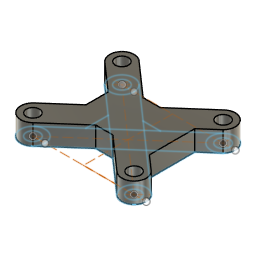
Drone v0 (Autodesk Fusion 360 design; units mm, degrees)
Autodesk Fusion 360 part; units mm, degrees
sketch "Skizze1" plane through (0, 0, 0) normal (0, 0, 1) x (1, 0, 0)
  line L0 (-50, 40) -> (0, 40) construction
  circle A0 centre (-50, 40) radius 3.25
  circle A1 centre (0, 40) radius 3.25
  line L1 (-25, 40) -> (-25, -4) construction
  line L2 (-25, -4) -> (0, -4) construction
  line L3 (0, -4) -> (-50, -4) construction
  circle A2 centre (-50, -4) radius 3.25
  circle A3 centre (0, -4) radius 3.25
  circle A4 centre (-50, 40) radius 6
  circle A5 centre (0, 40) radius 6
  circle A6 centre (0, -4) radius 6
  circle A7 centre (-50, -4) radius 6
  line L4 (-50, -4) -> (0, 40) construction
  line L5 (0, -4) -> (-50, 40) construction
  line L6 (-50, 40) -> (-50, 46) construction
  line L7 (-50, 40) -> (-49.8093, 40.2167) construction
  line L8 (-50, 40) -> (-45.7574, 44.2426) construction
  line L9 (-50, 40) -> (-44, 40) construction
  line L10 (-50, 40) -> (-56, 40) construction
  line L11 (-50, 40) -> (-54.2426, 35.7574) construction
  line L12 (0, -4) -> (6, -4) construction
  line L13 (0, -4) -> (4.2426, 0.2426) construction
  line L14 (0, -4) -> (6, -4) construction
  line L15 (0, -4) -> (0, -10) construction
  line L16 (0, -4) -> (-4.2426, -8.2426) construction
  line L17 (-4.2426, -8.2426) -> (-54.2426, 35.7574)
  line L18 (4.2426, 0.2426) -> (-45.7574, 44.2426)
  line L19 (0, 40) -> (0, 46) construction
  line L20 (0, 40) -> (-4.2426, 44.2426) construction
  line L21 (0, 40) -> (4.2426, 35.7574) construction
  line L22 (0, 40) -> (6, 40) construction
  line L23 (-50, -4) -> (-45.7574, -8.2426) construction
  line L24 (-50, -4) -> (-44, -4) construction
  line L25 (-50, -4) -> (-54.2426, 0.2426) construction
  line L26 (-50, -4) -> (-44, -4) construction
  line L27 (-54.2426, 0.2426) -> (-4.2426, 44.2426)
  line L28 (4.2426, 35.7574) -> (-45.7574, -8.2426)
  line L29 (-3.2166, 6.8068) -> (-3.2166, 29.1932)
  line L30 (-40.3073, 12.5057) -> (-40.3073, 23.4943)
  line L31 (-20.7574, 6.2903) -> (-29.2426, 6.2903)
  line L32 (-20.7574, 29.7097) -> (-29.2426, 29.7097)
  dimension "d2" = 6.5
  dimension "d3" = 6.5
  dimension "d4" = 6.5
  dimension "d5" = 6.5
  dimension "d6" = 12
  dimension "d7" = 12
  dimension "d8" = 12
  dimension "d9" = 45
  dimension "d10" = 135
  dimension "d11" = 6
  dimension "d12" = 45
  dimension "d13" = 135
  dimension "d14" = 135
  dimension "d15" = 45
  dimension "d16" = 6
  dimension "d17" = 45
  dimension "d18" = 135
  constraint horizontal L0
  constraint coincident L0.start A0.centre
  constraint coincident L0.end A1.centre
  constraint midpoint L0 L1.start
  constraint perpendicular L0 L1
  constraint perpendicular L1 L2
  constraint perpendicular L1 L3
  constraint coincident L3.end A2.centre
  constraint coincident L2.end L3.start
  constraint concentric A0 A4
  constraint concentric A1 A5
  constraint concentric A3 A6
  constraint concentric A2 A7
  constraint coincident A4 L6.end
  constraint vertical L6
  constraint perpendicular L5 L7
  constraint horizontal L9
  constraint coincident A4 L10.end
  constraint horizontal L10
  constraint coincident A6 L12.end
  constraint parallel L2 L12
  constraint horizontal L14
  constraint coincident A6 L15.end
  constraint vertical L15
  constraint coincident A5 L19.end
  constraint perpendicular L0 L19
  constraint horizontal L22
  constraint horizontal L24
  constraint horizontal L26
  constraint parallel L27 L28
  constraint coincident L18 L29.start
  constraint coincident L28 L29.end
  constraint vertical L29
  constraint coincident L27 L30.start
  constraint coincident L17 L30.end
  constraint parallel L29 L30
  constraint coincident L17 L31.start
  constraint coincident L28 L31.end
  constraint perpendicular L1 L31
  constraint coincident L27 L32.start
  constraint coincident L18 L32.end
  constraint perpendicular L1 L32
  measures "d2" diameter of A0
  measures "d3" diameter of A1
  measures "d4" diameter of A2
  measures "d5" diameter of A3
  measures "d6" diameter of A5
  measures "d7" diameter of A6
  measures "d8" diameter of A7
  measures "d9" angle of L8 L9
  measures "d10" angle of L10 L11
  measures "d11" distance of L2.end L13.end
  measures "d12" angle of L13 L14
  measures "d13" angle of L15 L16
  measures "d14" angle of L19 L20
  measures "d15" angle of L21 L22
  measures "d16" distance of L3.end L23.end
  measures "d17" angle of L23 L24
  measures "d18" angle of L25 L26
extrude "Extrusion1" add sketch "Skizze1" along normal blind 10 contours A4 L17 | A4 L17 L18 L27 | A5 L18 L27 L28 | L17 L18 L27 L28 | A7 L17 L27 L28 | A6 L17 L18 L28 | A5 L28 | A7 L27 | A6 L18 picked at (-55.035, 39.3919) picked at (-3.2811, 43.8676) picked at (-46.7227, -7.8704) picked at (-3.2811, -7.8676)
extrude "Extrusion2" add sketch "Skizze1" along normal blind 10 contours L18 L27 L32 | L17 L27 L30 | L18 L28 L29 | L17 L28 L31
